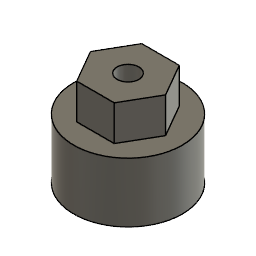
clamp_coupler_6mm_v0_1 (Autodesk Fusion 360 design; units mm, degrees)
part number: 2026-05-27-20-20-33-516
Autodesk Fusion 360 part; units mm, degrees
cylinder "圆柱体基本要素1" add diameter 20 height 11 placed x (1, 0, 0) y (0, 0, -1) z (0, 1, 0) at (0, 0, 0)
sketch "草图2" plane through (0, 11, 0) normal (0, 1, 0) x (-1, 0, 0)
  circle A0 centre (0, 0) radius 10
  line L0 (3.4641, -6) -> (-3.4641, -6)
  line L1 (-3.4641, -6) -> (-6.9282, 0)
  line L2 (-6.9282, 0) -> (-3.4641, 6)
  line L3 (-3.4641, 6) -> (3.4641, 6)
  line L4 (3.4641, 6) -> (6.9282, 0)
  line L5 (6.9282, 0) -> (3.4641, -6)
  line L6 (3.4641, -6) -> (-3.4641, 6) construction
  dimension "d4" = 12
  dimension "d5" = 120
  dimension "d6" = 120
  constraint horizontal L0
  constraint parallel L0 L3
  constraint parallel L1 L4
  constraint parallel L2 L5
  constraint equal L0 L1
  constraint equal L1 L2
  constraint equal L1 L3
  constraint equal L1 L4
  constraint midpoint L6 A0.centre
  constraint coincident A0.centre origin
  measures "d4" distance of L0 L3
  measures "d5" angle of L0 L5
  measures "d6" angle of L1 L2
extrude "拉伸1" add sketch "草图2" along normal blind 6.5 contours L0 L1 L2 L3 L4 L5
cylinder "圆柱体基本要素2" cut diameter 4 height -5.7 placed x (1, 0, 0) y (0, 0, -1) z (0, 1, 0) at (0, 17.5, 0)
cylinder "圆柱体基本要素3" cut diameter 6 height -11.8 placed x (1, 0, 0) y (0, 0, -1) z (0, 1, 0) at (0, 11.8, 0)
